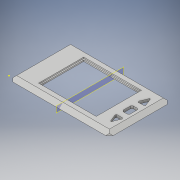
# Autodesk Inventor part: TopCover
Saved by Autodesk Inventor 2019 (Build 230136000, 136)
## iProperties
Created: 2021-04-26
Part Number: TopCover
Material: Všeobecné
Document SubType Name: Modeling
Designer: miko flosso
Density: 1 g/cm^3
Appearance: Výchozí
Author: miko flosso
Autodesk Inventor part; units mm, degrees
ref_plane "YZ Plane" through (0, 0, 0) normal (1, 0, 0) x (0, 1, 0)
ref_plane "XZ Plane" through (0, 0, 0) normal (0, 1, 0) x (-1, 0, 0)
sketch "Náčrt1" plane through (0, 0, 0) normal (0, 1, 0) x (-1, 0, 0)
  line L0 (0, 0) -> (-80, 0)
  line L1 (-80, 0) -> (-80, -49)
  line L2 (-80, -49) -> (0, -49)
  line L3 (0, -49) -> (0, 0)
  dimension "d0" = 80
  dimension "d1" = 49
  constraints: 8 end point, 2 parallel, 1 horizontal, 1 perpendicular
  measures "d0" distance of L2.end L1.end
  measures "d1" distance of L1.end L0.end
extrude "Vysunutí1" add sketch "Náčrt1" along normal blind 3
chamfer "Zkosení1" distance 3 angle 45 4 edges at (0, 1.5, 0) (0, 1.5, -49) (80, 1.5, -49) (80, 1.5, 0)
chamfer "Zkosení2" distance 3 angle 45 4 edges at (40, 3, 0) (0, 3, -24.5) (40, 3, -49) (80, 3, -24.5)
sketch "Náčrt2" plane through (0, 3, 0) normal (0, 1, 0) x (1, 0, 0)
  line L0 (18, 41.5) -> (62, 41.5)
  line L1 (62, 41.5) -> (62, 7.5)
  line L2 (62, 7.5) -> (18, 7.5)
  line L3 (18, 7.5) -> (18, 41.5)
  line L4 (77, 49) -> (3, 49) projected
  line L5 (0, 46) -> (0, 3) projected
  point P0 (0, 0)
  dimension "d11" = 44
  dimension "d12" = 34
  dimension "d13" = 7.5
  dimension "d14" = 18
  constraints: 8 end point, 2 parallel, 1 horizontal, 1 perpendicular
  measures "d11" distance of L1.end L2.end
  measures "d12" distance of L0.end L1.end
  measures "d13" distance between parallel lines of L0 L4
  measures "d14" distance between parallel lines of L3 L5
extrude "Vysunutí2" cut sketch "Náčrt2" against normal blind 2.5
sketch "Náčrt3" plane through (0, 3, 0) normal (0, 1, 0) x (1, 0, 0)
  line L0 (63, 42.5) -> (17, 42.5)
  line L1 (17, 42.5) -> (17, 6.5)
  line L2 (17, 6.5) -> (63, 6.5)
  line L3 (63, 6.5) -> (63, 42.5)
  line L4 (63, 42.5) -> (17, 6.5) construction
  line L5 (17, 42.5) -> (63, 6.5) construction
  point P0 (0, 0)
  point P1 (40, 24.5)
  dimension "d17" = 46
  dimension "d18" = 36
  constraints: 12 end point, 2 midpoint, 2 parallel, 1 horizontal, 1 perpendicular
  measures "d17" distance of L2.end L1.end
  measures "d18" distance of L1.end L0.end
extrude "Vysunutí3" cut sketch "Náčrt3" against normal blind 1
sketch "Náčrt4" plane through (0, 3, 0) normal (0, 1, 0) x (1, 0, 0)
  line L0 (75.5, 16) -> (69, 16)
  line L1 (69, 16) -> (72.25, 8)
  line L2 (75.5, 16) -> (72.25, 8)
  line L3 (3, 0) -> (77, 0) projected
  line L4 (0, 46) -> (0, 3) projected
  point P0 (0, 0)
  dimension "d21" = 6.5
  constraints: 6 end point
  measures "d21" distance of L0.end L0.start
extrude "Vysunutí4" cut sketch "Náčrt4" against normal blind 2.5
chamfer "Zkosení3" distance 1 angle 45 3 edges at (69, 1.75, -16) (75.5, 1.75, -16) (72.25, 1.75, -8)
ref_plane "Pracovní rovina1" through (77, 0, -24.5) normal (0, 0, -1) x (-1, 0, 0)
mirror "Zrcadlit1" about plane through (77, 0, -24.5) normal (0, 0, -1) of "Vysunutí4", "Zkosení3"
sketch "Náčrt5" plane through (0, 3, 0) normal (0, 1, 0) x (1, 0, 0)
  line L0 (69.3705, 20.5) -> (74.8705, 20.5)
  line L1 (74.8705, 20.5) -> (74.8705, 28.5)
  line L2 (74.8705, 28.5) -> (69.3705, 28.5)
  line L3 (69.3705, 28.5) -> (69.3705, 20.5)
  line L4 (3, 0) -> (77, 0) projected
  point P0 (0, 0)
  dimension "d30" = 5.5
  dimension "d31" = 8
  dimension "d32" = 20.5
  constraints: 8 end point, 2 parallel, 1 horizontal, 1 perpendicular
  measures "d30" distance of L2.end L1.end
  measures "d31" distance of L1.end L0.end
  measures "d32" distance between parallel lines of L4 L0
extrude "Vysunutí5" cut sketch "Náčrt5" against normal blind 2.5
chamfer "Zkosení4" distance 1 angle 45 4 edges at (69.3705, 1.75, -28.5) (69.3705, 1.75, -20.5) (74.8705, 1.75, -20.5) (74.8705, 1.75, -28.5)
sketch "Náčrt6" plane through (0, 3, 0) normal (0, 1, 0) x (1, 0, 0)
  point P0 (0, 0)
sketch "Náčrt7" plane through (0, 0, 0) normal (0, -1, 0) x (1, 0, 0)
  line L0 (3.8284, -2) -> (76.1716, -2)
  line L1 (77.9939, -3.8223) -> (77.9939, -45.1777)
  line L2 (76.2085, -46.9631) -> (3.9251, -46.9631)
  line L3 (2, -46) -> (2, -3.8284)
  line L4 (3, 0) -> (77, 0) projected
  line L5 (0, -46) -> (0, -3) projected
  line L6 (0, -46) -> (2.8284, -46) construction
  line L7 (2, -45.0688) -> (3.9251, -46.9631)
  line L8 (3, -49) -> (0, -46) projected
  line L9 (80, -46) -> (77, -49) projected
  line L10 (80, -46) -> (82.8284, -46) construction
  line L11 (77.9939, -45.1777) -> (76.2085, -46.9631)
  line L12 (77, 0) -> (80, -3) projected
  line L13 (76.1716, -2) -> (77.9939, -3.8223)
  line L14 (2, -3.8284) -> (3.8284, -2)
  line L15 (0, -3) -> (3, 0) projected
  point P0 (0, 0)
  dimension "d40" = 2
  dimension "d41" = 2
  dimension "d43" = 2
  dimension "d45" = 2
  dimension "d46" = 2
  dimension "d47" = 2
  constraints: 20 end point, 3 horizontal, 2 parallel, 2 point on line, 1 perpendicular
  measures "d40" distance between parallel lines of L4 L0
  measures "d41" distance between parallel lines of L5 L3
  measures "d43" distance from line of L6.end L8
  measures "d45" distance between parallel lines of L9 L11
  measures "d46" distance between parallel lines of L13 L12
  measures "d47" distance between parallel lines of L14 L15
extrude "Vysunutí6" cut sketch "Náčrt7" against normal blind 1
sketch "Náčrt8" plane through (77.9939, 0, -45.1777) normal (-1, 0, 0) x (0, 0, 1)
  line L0 (1.7879, 1) -> (1.7879, -1.5)
  line L1 (1.7879, -1.5) -> (39.5674, -1.5)
  line L2 (39.5674, -1.5) -> (39.5674, 1)
  line L3 (41.3554, 1) -> (0, 1) projected
  line L4 (39.5674, 1) -> (1.7879, 1)
  point P0 (45.1777, 0)
  constraints: 8 end point, 2 point on line, 1 parallel
extrude "Vysunutí7" add sketch "Náčrt8" along normal blind 1
chamfer "Zkosení5" distance 1.5 angle 45 2 edges at (77.4939, -1.5, -5.6103) (77.4939, -1.5, -43.3897)
sketch "Náčrt9" plane through (77.9939, 0, -45.1777) normal (1, 0, 0) x (0, 0, -1)
  line L0 (-3.2879, -1.5) -> (-3.2879, 0)
  line L1 (-3.2879, -1.5) -> (-38.0674, -1.5) projected
  line L2 (-3.2879, -1.5) -> (-38.0674, -1.5)
  line L3 (-38.0674, -1.5) -> (-38.0674, 0)
  line L4 (-42.1777, 0) -> (0.8223, 0) projected
  point P0 (-45.1777, 0)
  point P1 (-1.7879, 0)
  constraints: 6 end point, 1 horizontal, 1 perpendicular, 1 point on line, 1 vertical
extrude "Vysunutí8" add sketch "Náčrt9" along normal blind 0.5 draft -80
ref_plane "Pracovní rovina2" through (39.9969, 0, -45.1777) normal (-1, 0, 0) x (0, 0, 1)
mirror "Zrcadlit2" about plane through (39.9969, 0, -45.1777) normal (-1, 0, 0) of "Vysunutí7", "Zkosení5", "Vysunutí8"
